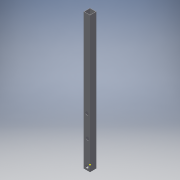
# Autodesk Inventor part: AP 2
Saved by Autodesk Inventor 2016 (Build 200138000, 138)
## iProperties
Created: 2016-02-17
Part Number: AP 2
Material: Generic
Document SubType Name: Modeling
Designer: Admin
Density: 1 g/cm^3
Appearance: Default
Author: Admin
Autodesk Inventor part; units mm, degrees
ref_plane "YZ Plane" through (0, 0, 0) normal (1, 0, 0) x (0, 1, 0)
ref_plane "XZ Plane" through (0, 0, 0) normal (0, 1, 0) x (-1, 0, 0)
ref_plane "XY Plane" through (0, 0, 0) normal (0, 0, 1) x (1, 0, 0)
sketch "Sketch1" plane through (0, 0, 0) normal (0, 1, 0) x (-1, 0, 0)
  line L0 (0, 0) -> (25.4, 0)
  line L1 (25.4, 0) -> (25.4, -25.4)
  line L2 (25.4, -25.4) -> (0, -25.4)
  line L3 (0, -25.4) -> (0, 0)
  line L4 (23.8125, -23.8125) -> (23.8125, -1.5875)
  line L5 (23.8125, -1.5875) -> (1.5875, -1.5875)
  line L6 (1.5875, -1.5875) -> (1.5875, -23.8125)
  line L7 (1.5875, -23.8125) -> (23.8125, -23.8125)
  dimension "d0" = 25.4
  dimension "d1" = 25.4
  dimension "d2" = 1.5875
  constraints: 16 end point, 4 parallel, 2 perpendicular, 1 horizontal, 3 other
  measures "d0" distance of L1.end L2.end
  measures "d1" distance of L0.end L1.end
  measures "d2" distance between parallel lines of L1 L4
extrude "Extrusion1" add sketch "Sketch1" along normal blind 419.1
sketch "Sketch3" plane through (-25.4, 0, 0) normal (0, 0, 1) x (1, 0, 0)
  point P0 (25.4, 0)
sketch "Sketch4" plane through (-25.4, 0, 0) normal (0, 0, 1) x (1, 0, 0)
  circle A0 centre (12.7, 406.4) radius 6.35
  line L0 (25.4, 0) -> (0, 0) projected
  line L1 (25.4, 0) -> (25.4, 419.1) projected
  line L2 (1.5875, 419.1) -> (23.8125, 419.1) projected
  dimension "d8" = 12.7
  dimension "d28" = 12.7
  dimension "d29" = 12.7
  constraints: 1 centre point
  measures "d8" diameter of A0
  measures "d28" distance from line of L1 A0.centre
  measures "d29" distance from line of L2 A0.centre
extrude "Extrusion3" cut sketch "Sketch4" against normal blind 25.4
sketch "Sketch5" plane through (-25.4, 0, 0) normal (0, 0, 1) x (1, 0, 0)
  circle A0 centre (12.7, 266.7) radius 6.35
  line L0 (25.4, 0) -> (0, 0) projected
  dimension "d12" = 12.7
  dimension "d15" = 266.7
  constraints: 1 centre point
  measures "d12" diameter of A0
  measures "d15" distance from line of L0 A0.centre
extrude "Extrusion4" cut sketch "Sketch5" against normal blind 25.4
sketch "Sketch7" plane through (0, 0, 0) normal (0, -1, 0) x (1, 0, 0)
  line L0 (0, 0) -> (-25.4, 0)
  line L1 (-25.4, 0) -> (-25.4, -25.4)
  line L2 (-25.4, -25.4) -> (0, -25.4)
  line L3 (0, -25.4) -> (0, 0)
  line L4 (-1.5875, -23.8125) -> (-23.8125, -23.8125) projected
  line L5 (-23.8125, -1.5875) -> (-1.5875, -1.5875) projected
  line L6 (-23.8125, -23.8125) -> (-1.5875, -23.8125)
  line L7 (-1.5875, -23.8125) -> (-1.5875, -1.5875)
  line L8 (-1.5875, -1.5875) -> (-23.8125, -1.5875)
  line L9 (-23.8125, -1.5875) -> (-23.8125, -23.8125)
  constraints: 16 end point, 4 parallel, 2 horizontal, 2 perpendicular
extrude "Extrusion6" add sketch "Sketch7" along normal blind 25.4
sketch "Sketch8" plane through (-25.4, 419.1, 0) normal (0, 0, 1) x (1, 0, 0)
  circle A0 centre (12.7, -431.8) radius 6.35
  line L0 (25.4, -444.5) -> (25.4, 0) projected
  line L1 (25.4, -444.5) -> (0, -444.5) projected
  point P0 (25.4, -419.1)
  dimension "d23" = 12.7
  dimension "d24" = 12.7
  dimension "d27" = 12.7
  constraints: 1 centre point
  measures "d23" diameter of A0
  measures "d24" distance from line of L0 A0.centre
  measures "d27" distance from line of L1 A0.centre
extrude "Extrusion7" cut sketch "Sketch8" against normal blind 25.4
body "Solid1"
